Autodesk Fusion 360 part; units mm, degrees
(part 2 of 2)
sketch "スケッチ4" plane through (0, 0, 2) normal (0, 0, 1) x (-1, 0, 0)
  line L0 (-9, -13) -> (-9, -15)
  line L1 (-9, -15) -> (9, -15)
  line L2 (9, -15) -> (9, -13)
  line L3 (9, -13) -> (27, -13)
  line L4 (27, -13) -> (27, -15)
  line L5 (27, -15) -> (45, -15)
  line L6 (45, -15) -> (45, -9)
  line L7 (45, -9) -> (47, -9)
  line L8 (47, -9) -> (47, -3)
  line L9 (47, -3) -> (45, -3)
  line L10 (45, -3) -> (45, 3)
  line L11 (45, 3) -> (47, 3)
  line L12 (47, 3) -> (47, 9)
  line L13 (47, 9) -> (45, 9)
  line L14 (45, 9) -> (45, 15)
  line L15 (45, 15) -> (27, 15)
  line L16 (27, 15) -> (27, 13)
  line L17 (27, 13) -> (9, 13)
  line L18 (9, 13) -> (9, 15)
  line L19 (9, 15) -> (-9, 15)
  line L20 (-9, 15) -> (-9, 13)
  line L21 (-9, 13) -> (-27, 13)
  line L22 (-27, 13) -> (-27, 15)
  line L23 (-27, 15) -> (-45, 15)
  line L24 (-45, 15) -> (-45, 9)
  line L25 (-45, 9) -> (-47, 9)
  line L26 (-47, 9) -> (-47, 3)
  line L27 (-47, 3) -> (-45, 3)
  line L28 (-45, 3) -> (-45, -3)
  line L29 (-45, -3) -> (-47, -3)
  line L30 (-47, -3) -> (-47, -9)
  line L31 (-47, -9) -> (-45, -9)
  line L32 (-45, -9) -> (-45, -15)
  line L33 (-45, -15) -> (-27, -15)
  line L34 (-27, -15) -> (-27, -13)
  line L35 (-27, -13) -> (-9, -13)
  line L36 (38, 11) -> (-14, 11)
  line L37 (-14, 11) -> (-14, 1)
  line L38 (-14, 1) -> (38, 1)
  line L39 (38, 1) -> (38, 11)
  dimension "d23" = 2
  dimension "d24" = 10
  dimension "d25" = 52
  dimension "d26" = 7
  constraint horizontal L36
  constraint vertical L37
  constraint horizontal L38
  constraint vertical L39
  measures "d23" distance of L17 L36
  measures "d24" distance of L36.start L38.end
  measures "d25" distance of L37.end L38.end
  measures "d26" distance of L14 L39
extrude "押し出し4" cut sketch "スケッチ4" against normal up to surface (2 mm away) contours L36 L37 L38 L39
equation "d3 = t"
equation "t = 2 mm" comment "板厚"
equation "d6 = t"
equation "w = 11.6 mm" comment "かみ合い幅"
equation "d9 = w3"
equation "d10 = w3 / 2"
equation "w2 = 18 mm"
equation "w3 = 6 mm"
equation "d16 = w2"
equation "d21 = t"
equation "d22 = w2 / 2"
